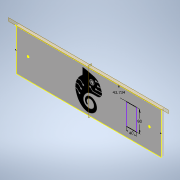
# Autodesk Inventor part: wooden_backcover
Saved by Autodesk Inventor 2020 (Build 240168000, 168)
## iProperties
Created: 2019-07-26
Part Number: wooden_backcover
Material: Generic
Document SubType Name: Modeling
Designer: erwin
Density: 1 g/cm^3
Appearance: Default
Mass: 1273.68 g
Surface Area: 2310.96 cm^2
Volume: 1273.68 cm^3
Author: erwin
Autodesk Inventor part; units mm, degrees
ref_plane "YZ Plane" through (0, 0, 0) normal (1, 0, 0) x (0, 1, 0)
ref_plane "XZ Plane" through (0, 0, 0) normal (0, 1, 0) x (-1, 0, 0)
ref_plane "XY Plane" through (0, 0, 0) normal (0, 0, 1) x (1, 0, 0)
ref_plane "Work Plane1" through (0, 0, 0) normal (0, 0, 1) x (1, 0, 0)
sketch "Sketch1" plane through (0, 0, 0) normal (0, 0, 1) x (1, 0, 0)
  line L0 (612, -44.7721) -> (612, -100.7605) projected
  line L1 (0, 0) -> (612, 0) projected
  line L2 (612, -176) -> (0, -176) projected
  line L3 (612, 0) -> (0, 0)
  line L4 (0, 0) -> (0, -176)
  line L5 (0, -176) -> (612, -176)
  line L6 (612, -176) -> (612, 0)
  constraints: 8 end point, 2 parallel, 1 horizontal, 1 perpendicular
extrude "Extrusion1" add sketch "Sketch1" against normal blind 12
thicken "Thicken1" operation add thickness 1 both sides no extend neighbours yes toward (1, 0, 0) faces at (0, -58.6667, -4) (204, -176, -4) (612, -29.8481, -4) (612, -82.0977, -4) (612, -150.9202, -4) (408, 0, -4)
sketch "Sketch2" plane through (0, 0, 0) normal (0, 0, 1) x (1, 0, 0)
  circle A0 centre (51, -88) radius 4
  line L0 (611, -1) -> (1, -1) projected
  line L1 (1, -175) -> (611, -175) projected
  line L2 (1, -1) -> (1, -175) projected
  point P0 (0, 0)
  dimension "d4" = 8
  dimension "d5" = 87
  dimension "d6" = 87
  dimension "d7" = 50
  constraints: 1 centre point
  measures "d4" diameter of A0
  measures "d5" distance from line of L0 A0.centre
  measures "d6" distance from line of L1 A0.centre
  measures "d7" distance from line of L2 A0.centre
extrude "Extrusion2" cut sketch "Sketch2" against normal blind 12
ref_plane "Work Plane2" through (306, -175, 0) normal (-1, 0, 0) x (0, 0, 1)
mirror "Mirror1" about plane through (306, -175, 0) normal (-1, 0, 0) of "Extrusion2"
sketch "Sketch3" plane through (0, 0, 0) normal (0, 0, 1) x (1, 0, 0)
  line L0 (1, -1) -> (611, -1) construction
  line L1 (611, -1) -> (611, -175) construction
  line L2 (611, -175) -> (1, -175) construction
  line L3 (1, -175) -> (1, -1) construction
  line L4 (611, -175) -> (611, -1) projected
  line L5 (1, -1) -> (1, -175) projected
  point P0 (0, 0)
  point P1 (611, -88)
  point P2 (1, -88)
  constraints: 4 midpoint, 1 point on line, 2 other
sketch "Sketch5" plane through (0, 0, 0) normal (0, 0, 1) x (1, 0, 0)
  line L0 (486, -43) -> (506, -43)
  line L1 (516, -53) -> (516, -123)
  line L2 (506, -133) -> (486, -133)
  line L3 (476, -123) -> (476, -53)
  line L4 (611, -1) -> (1, -1) projected
  line L5 (1, -175) -> (611, -175) projected
  line L6 (611, -175) -> (611, -1) projected
  arc A0 (486, -43) -> (476, -53) centre (486, -53) ccw
  arc A1 (506, -133) -> (516, -123) centre (506, -123) ccw
  arc A2 (476, -123) -> (486, -133) centre (486, -123) ccw
  arc A3 (516, -53) -> (506, -43) centre (506, -53) ccw
  point P0 (0, 0)
  point P1 (516, -133)
  point P2 (516, -43)
  point P3 (476, -133)
  dimension "d10" = 40
  dimension "d11" = 90
  dimension "d12" = 42
  dimension "d13" = 42
  dimension "d14" = 95
  dimension "d15" = 10
  constraints: 8 end point, 8 point on circle, 8 tangent, 6 point on line, 4 centre point, 3 equal radius, 2 parallel, 1 horizontal, 1 perpendicular
  measures "d10" distance of point (516, -133) point (476, -133)
  measures "d11" distance of point (516, -43) point (516, -133)
  measures "d12" distance between parallel lines of L4 L0
  measures "d13" distance between parallel lines of L5 L2
  measures "d14" distance between parallel lines of L6 L1
  measures "d15" radius of A0
extrude "Extrusion3" cut sketch "Sketch5" against normal through all
mirror "Mirror2" about plane through (306, -175, 0) normal (-1, 0, 0) of "Extrusion3"
sketch "Sketch6" plane through (0, 0, 0) normal (0, 0, 1) x (1, 0, 0)
  point P0 (0, 0)
equation "\"d5\" = d6"
equation "\"d12\" = d13"
body "Solid1"
